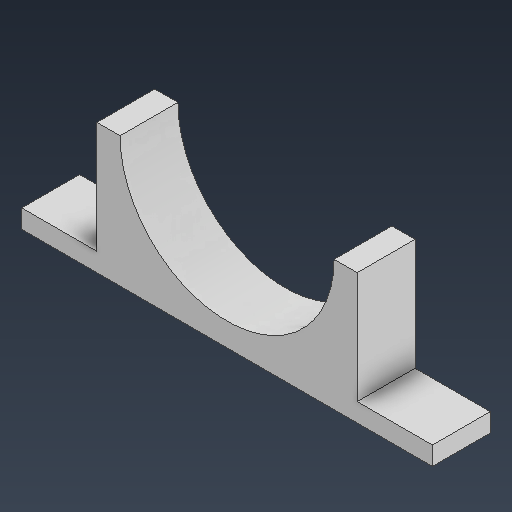
# Autodesk Inventor part: мотор подьем крепл 25-26
Saved by Autodesk Inventor 2025 (Build 290162000, 162)
## iProperties
Created: 2025-09-25
Part Number: мотор подьем крепл 25-26
Material: Типовые
Document SubType Name: Modeling
Designer: GameHD
Density: 1 g/cm^3
Appearance: По умолчанию
Author: GameHD
Autodesk Inventor part; units mm, degrees
ref_plane "YZ Plane" through (0, 0, 0) normal (1, 0, 0) x (0, 1, 0)
ref_plane "XZ Plane" through (0, 0, 0) normal (0, 1, 0) x (-1, 0, 0)
ref_plane "XY Plane" through (0, 0, 0) normal (0, 0, 1) x (1, 0, 0)
sketch "Эскиз1" plane through (0, 0, 0) normal (0, 0, 1) x (1, 0, 0)
  circle A0 centre (0, 0) radius 18.5
  circle A1 centre (0, 0) radius 22.5
  line L0 (-22.5, 0) -> (22.5, 0)
  line L1 (-22.5, 0) -> (-22.5, -22.5)
  line L2 (-22.5, -22.5) -> (-35.5, -22.5)
  line L3 (-35.5, -22.5) -> (-35.5, -19.3)
  line L4 (-35.5, -19.3) -> (-22.5, -19.3)
  line L5 (0, 0) -> (0, -7.9375)
  line L6 (22.5, 0) -> (22.5, -22.5)
  line L7 (22.5, -22.5) -> (35.5, -22.5)
  line L8 (35.5, -22.5) -> (35.5, -19.3)
  line L9 (35.5, -19.3) -> (22.5, -19.3)
  line L10 (-22.5, -22.5) -> (22.5, -22.5)
  point P0 (-18.5, 0)
  point P1 (18.5, 0)
  dimension "d0" = 37
  dimension "d1" = 45
  dimension "d2" = 13
  dimension "d3" = 3.2
  dimension "d4" = 13
  constraints: 22 end point, 4 symmetric about line, 3 perpendicular, 2 centre point, 2 coincident, 2 horizontal, 2 point on circle, 1 collinear, 1 tangent, 1 vertical
  measures "d0" diameter of A0
  measures "d1" diameter of A1
  measures "d2" distance of L1.end L2.end
  measures "d3" distance of L2.end L3.end
  measures "d4" distance of L3.end L4.end
extrude "Выдавливание1" add sketch "Эскиз1" along normal blind 10 contours L0 A1 A0 | L6 L10 A1 | A1 L10 L1 | L9 L8 L7 L6 | L1 L2 L3 L4 picked at (-20.9786, -1.6689)
